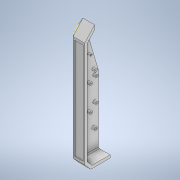
# Autodesk Inventor part: błotnik_v2
Saved by Autodesk Inventor 2022 (Build 260153000, 153)
## iProperties
Created: 2022-10-25
Part Number: błotnik_v2
Material: Generic
Document SubType Name: Modeling
Designer: Kamil
Density: 1 g/cm^3
Appearance: Default
Author: Kamil
Autodesk Inventor part; units mm, degrees
ref_plane "YZ Plane" through (0, 0, 0) normal (1, 0, 0) x (0, 1, 0)
ref_plane "XZ Plane" through (0, 0, 0) normal (0, 1, 0) x (-1, 0, 0)
ref_plane "XY Plane" through (0, 0, 0) normal (0, 0, 1) x (1, 0, 0)
sketch "Sketch1" plane through (0, 0, 0) normal (1, 0, 0) x (0, 1, 0)
  line L0 (-91.913208, 90.571897) -> (-91.913208, 0.571897)
  line L1 (-91.913208, 0.571897) -> (48.235078, 0.571897)
  arc A0 (48.235078, 0.571897) -> (67.938507, 0.571897) centre (58.086792, 2.287626) ccw
  line L2 (67.938507, 0.571897) -> (198.235078, 0.571897)
  arc A1 (198.235078, 0.571897) -> (217.938507, 0.571897) centre (208.086792, 2.287626) ccw
  line L3 (217.938507, 0.571897) -> (338.235078, 0.571897)
  arc A2 (338.235078, 0.571897) -> (357.938507, 0.571897) centre (348.086792, 2.287626) ccw
  line L4 (357.938507, 0.571897) -> (387.823998, 0.571897)
  arc A3 (387.823998, 0.571897) -> (392.823998, 1.911643) centre (387.823998, 10.571897) ccw
  line L5 (392.823998, 1.911643) -> (465.586792, 43.921262)
  arc A4 (465.586792, 43.921262) -> (453.086792, 90.571897) centre (453.086792, 65.571897) ccw
  line L6 (453.086792, 90.571897) -> (215.586792, 90.571897)
  arc A5 (215.586792, 90.571897) -> (200.586792, 90.571897) centre (208.086792, 90.571897) ccw
  line L7 (200.586792, 90.571897) -> (65.586792, 90.571897)
  arc A6 (65.586792, 90.571897) -> (50.586792, 90.571897) centre (58.086792, 90.571897) ccw
  line L8 (50.586792, 90.571897) -> (-91.913208, 90.571897)
  line L9 (394.423369, 30.080909) -> (384.836861, 44.460672)
  arc A7 (384.836916, 46.679556) -> (384.836861, 44.460672) centre (386.500961, 45.570073) ccw
  line L10 (384.836916, 46.679556) -> (394.426376, 61.062197)
  arc A8 (398.090422, 59.952509) -> (394.426376, 61.062197) centre (396.090422, 59.952714) ccw
  line L11 (398.090422, 59.952509) -> (398.08747, 31.190104)
  arc A9 (394.423369, 30.080909) -> (398.08747, 31.190104) centre (396.08747, 31.19031) ccw
  line L12 (46.086792, 47.681546) -> (11.958566, 47.681546)
  arc A10 (11.064139, 51.4704) -> (11.958566, 47.681546) centre (11.958566, 49.681546) ccw
  line L13 (11.064139, 51.4704) -> (45.192365, 68.534513)
  arc A11 (48.086792, 66.745659) -> (45.192365, 68.534513) centre (46.086792, 66.745659) ccw
  line L14 (48.086792, 66.745659) -> (48.086792, 49.681546)
  arc A12 (46.086792, 47.681546) -> (48.086792, 49.681546) centre (46.086792, 49.681546) ccw
  line L15 (278.981219, 39.534513) -> (319.328744, 19.360751)
  arc A13 (318.434316, 15.571897) -> (319.328744, 19.360751) centre (318.434316, 17.571897) ccw
  line L16 (318.434316, 15.571897) -> (237.739268, 15.571897)
  arc A14 (236.844841, 19.360751) -> (237.739268, 15.571897) centre (237.739268, 17.571897) ccw
  line L17 (236.844841, 19.360751) -> (277.192365, 39.534513)
  arc A15 (278.981219, 39.534513) -> (277.192365, 39.534513) centre (278.086792, 37.745659) ccw
  line L18 (367.833079, 75.571897) -> (388.344391, 75.571897)
  arc A16 (390.008437, 72.462414) -> (388.344391, 75.571897) centre (388.344391, 73.571897) ccw
  line L19 (390.008437, 72.462414) -> (379.752228, 57.079758)
  arc A17 (376.424082, 57.07984) -> (379.752228, 57.079758) centre (378.088183, 58.189241) ccw
  line L20 (376.424082, 57.07984) -> (366.168978, 72.462497)
  arc A18 (367.833079, 75.571897) -> (366.168978, 72.462497) centre (367.833079, 73.571897) ccw
  line L21 (361.750893, 61.061868) -> (371.338877, 46.679891)
  arc A19 (371.338822, 44.461008) -> (371.338877, 46.679891) centre (369.674777, 45.570491) ccw
  line L22 (371.338822, 44.461008) -> (361.750838, 30.080579)
  arc A20 (358.086792, 31.190063) -> (361.750838, 30.080579) centre (360.086792, 31.190063) ccw
  line L23 (358.086792, 31.190063) -> (358.086792, 59.952467)
  arc A21 (361.750893, 61.061868) -> (358.086792, 59.952467) centre (360.086792, 59.952467) ccw
  line L24 (89.12425, 75.571897) -> (177.049334, 75.571897)
  arc A22 (177.887451, 71.755978) -> (177.049334, 75.571897) centre (177.049334, 73.571897) ccw
  line L25 (177.887451, 71.755978) -> (133.924909, 51.465574)
  arc A23 (132.248676, 51.465574) -> (133.924909, 51.465574) centre (133.086792, 53.281493) ccw
  line L26 (132.248676, 51.465574) -> (88.286134, 71.755978)
  arc A24 (89.12425, 75.571897) -> (88.286134, 71.755978) centre (89.12425, 73.571897) ccw
  line L27 (-11.018781, 39.534513) -> (29.328744, 19.360751)
  arc A25 (28.434316, 15.571897) -> (29.328744, 19.360751) centre (28.434316, 17.571897) ccw
  line L28 (28.434316, 15.571897) -> (-52.260732, 15.571897)
  arc A26 (-53.155159, 19.360751) -> (-52.260732, 15.571897) centre (-52.260732, 17.571897) ccw
  line L29 (-53.155159, 19.360751) -> (-12.807635, 39.534513)
  arc A27 (-11.018781, 39.534513) -> (-12.807635, 39.534513) centre (-11.913208, 37.745659) ccw
  line L30 (117.220784, 43.755978) -> (70.924909, 22.388651)
  arc A28 (68.086792, 24.20457) -> (70.924909, 22.388651) centre (70.086792, 24.20457) ccw
  line L31 (68.086792, 24.20457) -> (68.086792, 66.939224)
  arc A29 (70.924909, 68.755143) -> (68.086792, 66.939224) centre (70.086792, 66.939224) ccw
  line L32 (70.924909, 68.755143) -> (117.220784, 47.387816)
  arc A30 (117.220784, 43.755978) -> (117.220784, 47.387816) centre (116.382668, 45.571897) ccw
  line L33 (-71.913208, 24.398135) -> (-71.913208, 66.745659)
  arc A31 (-69.018781, 68.534513) -> (-71.913208, 66.745659) centre (-69.913208, 66.745659) ccw
  line L34 (-69.018781, 68.534513) -> (-26.671256, 47.360751)
  arc A32 (-26.671256, 43.783043) -> (-26.671256, 47.360751) centre (-27.565684, 45.571897) ccw
  line L35 (-26.671256, 43.783043) -> (-69.018781, 22.60928)
  arc A33 (-71.913208, 24.398135) -> (-69.018781, 22.60928) centre (-69.913208, 24.398135) ccw
  line L36 (177.049334, 15.571897) -> (89.12425, 15.571897)
  arc A34 (88.286134, 19.387816) -> (89.12425, 15.571897) centre (89.12425, 17.571897) ccw
  line L37 (88.286134, 19.387816) -> (132.248676, 39.67822)
  arc A35 (133.924909, 39.67822) -> (132.248676, 39.67822) centre (133.086792, 37.862301) ccw
  line L38 (133.924909, 39.67822) -> (177.887451, 19.387816)
  arc A36 (177.049334, 15.571897) -> (177.887451, 19.387816) centre (177.049334, 17.571897) ccw
  line L39 (330.192365, 25.10928) -> (292.844841, 43.783043)
  arc A37 (292.844841, 47.360751) -> (292.844841, 43.783043) centre (293.739268, 45.571897) ccw
  line L40 (292.844841, 47.360751) -> (330.192365, 66.034513)
  arc A38 (333.086792, 64.245659) -> (330.192365, 66.034513) centre (331.086792, 64.245659) ccw
  line L41 (333.086792, 64.245659) -> (333.086792, 26.898135)
  arc A39 (330.192365, 25.10928) -> (333.086792, 26.898135) centre (331.086792, 26.898135) ccw
  line L42 (379.751656, 34.060723) -> (390.004607, 18.681297)
  arc A40 (388.340506, 15.571897) -> (390.004607, 18.681297) centre (388.340506, 17.571897) ccw
  line L43 (388.340506, 15.571897) -> (367.833501, 15.571897)
  arc A41 (366.169455, 18.68138) -> (367.833501, 15.571897) centre (367.833501, 17.571897) ccw
  line L44 (366.169455, 18.68138) -> (376.42351, 34.060806)
  arc A42 (379.751656, 34.060723) -> (376.42351, 34.060806) centre (378.087555, 32.951323) ccw
  line L45 (237.739268, 75.571897) -> (318.434316, 75.571897)
  arc A43 (319.328744, 71.783043) -> (318.434316, 75.571897) centre (318.434316, 73.571897) ccw
  line L46 (319.328744, 71.783043) -> (278.981219, 51.60928)
  arc A44 (277.192365, 51.60928) -> (278.981219, 51.60928) centre (278.086792, 53.398135) ccw
  line L47 (277.192365, 51.60928) -> (236.844841, 71.783043)
  arc A45 (237.739268, 75.571897) -> (236.844841, 71.783043) centre (237.739268, 73.571897) ccw
  line L48 (196.086792, 47.681546) -> (158.695156, 47.681546)
  arc A46 (157.85704, 51.497465) -> (158.695156, 47.681546) centre (158.695156, 49.681546) ccw
  line L49 (157.85704, 51.497465) -> (195.248676, 68.755143)
  arc A47 (198.086792, 66.939224) -> (195.248676, 68.755143) centre (196.086792, 66.939224) ccw
  line L50 (198.086792, 66.939224) -> (198.086792, 49.681546)
  arc A48 (196.086792, 47.681546) -> (198.086792, 49.681546) centre (196.086792, 49.681546) ccw
  line L51 (-52.260732, 75.571897) -> (28.434316, 75.571897)
  arc A49 (29.328744, 71.783043) -> (28.434316, 75.571897) centre (28.434316, 73.571897) ccw
  line L52 (29.328744, 71.783043) -> (-11.018781, 51.60928)
  arc A50 (-12.807635, 51.60928) -> (-11.018781, 51.60928) centre (-11.913208, 53.398135) ccw
  line L53 (-12.807635, 51.60928) -> (-53.155159, 71.783043)
  arc A51 (-52.260732, 75.571897) -> (-53.155159, 71.783043) centre (-52.260732, 73.571897) ccw
  line L54 (220.981219, 68.534513) -> (263.328744, 47.360751)
  arc A52 (263.328744, 43.783043) -> (263.328744, 47.360751) centre (262.434316, 45.571897) ccw
  line L55 (263.328744, 43.783043) -> (220.981219, 22.60928)
  arc A53 (218.086792, 24.398135) -> (220.981219, 22.60928) centre (220.086792, 24.398135) ccw
  line L56 (218.086792, 24.398135) -> (218.086792, 66.745659)
  arc A54 (220.981219, 68.534513) -> (218.086792, 66.745659) centre (220.086792, 66.745659) ccw
  circle A55 centre (208.086792, 2.287626) radius 2.5
  circle A56 centre (348.086792, 2.287626) radius 2.5
  circle A57 centre (243.086792, 8.071897) radius 2.5
  circle A58 centre (183.086792, 37.681546) radius 2.5
  circle A59 centre (23.086792, 37.681546) radius 2.5
  circle A60 centre (-81.913208, 83.071897) radius 2.5
  circle A61 centre (100.086792, 83.071546) radius 2.5
  circle A62 centre (260.086792, 83.071546) radius 2.5
  circle A63 centre (343.086792, 37.681546) radius 2.5
  circle A64 centre (348.086792, 83.071897) radius 2.5
  circle A65 centre (58.086792, 2.287626) radius 2.5
  circle A66 centre (-81.913208, 8.071897) radius 2.5
  line L57 (413.086792, 68.571897) -> (453.086792, 68.571897)
  arc A67 (453.086792, 62.571897) -> (453.086792, 68.571897) centre (453.086792, 65.571897) ccw
  line L58 (453.086792, 62.571897) -> (413.086792, 62.571897)
  arc A68 (413.086792, 68.571897) -> (413.086792, 62.571897) centre (413.086792, 65.571897) ccw
  line L59 (493.086792, 110.571897) -> (493.086792, -89.428103)
  line L60 (493.086792, -89.428103) -> (-191.913208, -89.428103)
  circle A69 centre (453.086792, 65.571897) radius 40
  circle A70 centre (-151.913208, 65.571897) radius 40
  line L61 (493.086792, -89.428103) -> (-191.913208, -89.428103)
  line L62 (-191.913208, -89.428103) -> (-191.913208, -23.428103)
  line L63 (-191.913208, -23.428103) -> (493.086792, -23.428103)
  line L64 (493.086792, -23.428103) -> (493.086792, -89.428103)
  line L65 (493.086792, -89.428103) -> (513.086792, -89.428103)
  line L66 (493.086792, 111.079815) -> (493.086792, -89.428103)
  line L67 (453.086792, 65.571897) -> (503.100187, 121.461612)
  line L68 (479.760603, 95.379745) -> (493.097508, 110.283669)
  line L69 (493.097508, 110.283669) -> (453.663093, 145.571897)
  line L70 (453.663093, 145.571897) -> (531.887738, 75.571897)
  line L71 (-151.913208, 65.571897) -> (-191.775038, 110.416456)
  line L72 (-178.487761, 95.46827) -> (-191.775038, 110.416456)
  line L73 (-191.775038, 110.416456) -> (-234.945881, 72.042373)
  line L74 (-234.945881, 72.042373) -> (-158.179562, 140.279101)
  line L75 (528.008583, -89.357621) -> (513.008583, -89.357621)
  line L76 (518.005904, 87.994176) -> (528.008583, 99.17212)
  line L77 (465.586792, 134.901872) -> (475.589471, 146.079815)
  line L78 (532.147616, 95.46827) -> (475.589471, 146.079815)
  line L79 (475.589471, 146.079815) -> (554.381712, 75.571897)
  line L80 (518.005904, 87.994176) -> (531.887738, 75.571897)
  line L81 (543.062687, 75.571897) -> (584.645568, 75.571897)
  line L82 (584.645568, 75.571897) -> (398.349618, 75.571897)
  line L83 (-158.179562, 140.279101) -> (-132.743704, 162.756041)
  line L84 (-226.991417, -89.357621) -> (-211.991417, -89.357621)
  line L85 (-250.129793, 130.571897) -> (-250.129793, 145.571897)
  line L86 (-191.913208, -89.428103) -> (-191.913208, 65.571897)
  line L87 (-191.913208, 110.293639) -> (-191.913208, 110.571897)
  line L88 (-191.913208, 110.293639) -> (-201.878665, 121.504778)
  line L89 (-201.888524, 121.496015) -> (-174.803157, 145.571897)
  line L90 (-201.888524, 121.496015) -> (-254.656636, 74.591027)
  line L91 (-211.913208, -4.093976) -> (-211.913208, 29.447632)
  line L92 (-191.913208, 29.447632) -> (-191.913208, -4.093976)
  line L93 (-226.913208, -4.093976) -> (-226.913208, 29.447632)
  line L94 (-211.913208, 29.447632) -> (-211.913208, -4.093976)
  line L95 (-226.913208, -4.093976) -> (-211.913208, -4.093976)
  line L96 (-211.913208, -4.093976) -> (-211.913208, 115.899208)
  line L97 (-211.913208, 115.899208) -> (-226.913208, 115.899208)
  line L98 (-226.913208, 115.899208) -> (-226.913208, -4.093976)
  line L99 (-226.913208, -4.093976) -> (-211.913208, -4.093976)
  line L100 (-211.913208, -4.093976) -> (-211.913208, -158.327462)
  line L101 (-211.913208, -158.327462) -> (-226.913208, -158.327462)
  line L102 (-226.913208, -158.327462) -> (-226.913208, -4.093976)
  line L103 (531.887738, 75.571897) -> (543.890953, 88.985429)
  line L104 (-191.913208, 110.293639) -> (-203.871757, 123.747006)
  line L105 (-211.913208, -4.093976) -> (-229.913208, -4.093976)
  line L106 (-229.913208, -4.093976) -> (-229.913208, 127.927783)
  line L107 (-229.913208, 127.927783) -> (-229.913208, -180.474457)
  line L108 (-203.871757, 123.747006) -> (-168.215619, 155.441351)
  line L109 (-168.215619, 155.441351) -> (-240.454048, 91.229415)
  line L110 (543.890953, 88.985429) -> (459.90651, 164.139633)
  line L111 (459.90651, 164.139633) -> (563.854127, 71.121209)
  circle A71 centre (348.086792, 83.071897) radius 6.710252
  circle A72 centre (-81.913208, 8.071897) radius 5.766352
  line L112 (-211.913208, -23.428103) -> (-229.913208, -23.428103)
  line L113 (493.086792, -23.428103) -> (732.784985, -23.428103)
  line L114 (558.880507, 75.571897) -> (222.333079, -23.428103)
  line L115 (222.333079, -23.428103) -> (-229.913208, -23.428103)
  line L116 (453.086792, 105.571897) -> (495.489419, 105.571897)
  line L117 (453.086792, 105.571897) -> (453.086792, 123.571897)
  line L118 (453.086792, 123.571897) -> (517.1971, 123.571897)
  line L119 (453.086792, 123.571897) -> (453.086792, 138.571897)
  line L120 (453.086792, 138.571897) -> (512.645416, 138.571897)
  line L121 (453.086792, 138.571897) -> (-211.913208, 138.571897)
  line L122 (453.086792, 123.571897) -> (-280.749903, 123.571897)
  point P0 (0, 0)
  point P1 (0, 0)
  point P2 (558.880507, 75.571897)
  point P3 (488.478326, 138.571897)
  point P4 (-187.193755, 138.571897)
  point P5 (-203.716104, 123.571897)
  point P6 (-204.068755, 123.571897)
  point P7 (-229.913208, 100.59905)
  point P8 (-211.913208, 92.515861)
  point P9 (-176.975167, 123.571897)
  point P10 (478.247981, 123.571897)
  point P11 (493.086792, 110.293259)
  point P12 (493.086792, 110.271694)
  dimension "d2" = 685
  dimension "d3" = 200
  dimension "d9" = 20
  dimension "d11" = 20
  dimension "d13" = 15
  dimension "d14" = 15
  dimension "d15" = 15
  dimension "d20" = 15
  dimension "d23" = 18
  dimension "d25" = 18
  dimension "d26" = 18
  dimension "d28" = 18
  dimension "d29" = 15
  constraints: 246 end point, 118 point on circle, 73 centre point, 26 point on line, 17 perpendicular, 12 parallel, 7 horizontal, 3 coincident, 3 tangent, 2 vertical, 1 collinear
  measures "d2" distance of L59.start L87.end
  measures "d3" distance of L59.start L59.end
  measures "d9" distance of L68.start L68.end
  measures "d11" distance of L71.end L72.start
  measures "d13" distance of L75.start L75.end
  measures "d14" distance of L76.start L76.end
  measures "d15" distance of L77.end L77.start
  measures "d20" distance of L87.start L88.end
  measures "d23" distance of L70.end L103.end
  measures "d25" distance of L87.start L104.end
  measures "d26" distance of L99.end L105.end
  measures "d28" distance of L116.start L117.end
  measures "d29" distance of L117.end L119.end
extrude "Extrusion1" add sketch "Sketch1" along normal blind 100 contours L119 L120 L69 L118 | L122 L74 L121 L119 | L118 L78 L67 L69 | L69 L77 L120 L78 L118 | L122 L89 L121 L74 | L74 L73 L88 L89 L122 | L112 L102 L95 L100 | L67 L78 L76 L70 | L69 L120 L77 | L118 L110 L103 L79 L78 | L78 L120 L110 L118 | L122 L104 L108 L121 L89 | L89 L104 L122 | L95 L93 L98 L73 L96 L91 | L112 L107 L105 L102 | L81 L79 L103 L111 | L103 L79 L81 L82 | L70 L76 L78 L79 L103 | L73 L96 L90 L89 L88 | L89 L90 L96 L97 L109 L122 L104 | L105 L106 L73 L98 L93 | L73 L98 L90 L96 | L73 L106 L90 L98 | L90 L98 L109 L97 L96 | L90 L106 L109 L98
extrude "Extrusion2" add sketch "Sketch1" against normal blind 20 contours L8 A6 L7 A5 L6 A69 L57 A68 L58 L114 L42 A42 L44 L3 A1 L2 A0 L1 L0 | L0 L1 A0 L2 A1 L3 L114 L63 L86 A70 L71 L74 L122 L117 A69 L6 A5 L7 A6 L8 | A69 L67 A4 L6 | L6 A4 L67 L82 A69 | L116 L67 A69 | L117 L118 L69 L59 L67 L116 | L82 L67 A67 L57 A69 | L44 A42 L42 L114 | L67 A69 L82 A4 | A4 L82 L67 | L67 L116 L59 L82 A69 | L67 L59 L116 | L119 L120 L69 L118 | L122 L74 L121 L119 | A69 L58 A68 L57 | L57 A67 L58 A69 | L82 A4 L114 A69 L58 A67 L67 | L115 L100 L91 L96 L73 L71 A70 L86 | L82 A69 L114 A4 | L82 L59 A69 | L67 L70 L82 L59 | L118 L78 L67 L69 | L69 L77 L120 L78 L118 | L122 L89 L121 L74 | L74 L73 L88 L89 L122 | L112 L102 L95 L100 | L114 A69 L59 | L59 L82 L81 L114 | L67 L78 L76 L70 | L69 L120 L77 | L118 L110 L103 L79 L78 | L78 L120 L110 L118 | L122 L104 L108 L121 L89 | L89 L104 L122 | L95 L93 L98 L73 L96 L91 | L112 L107 L105 L102 | L81 L79 L103 L111 | L103 L79 L81 L82 | L70 L76 L78 L79 L103 | A70 | L73 L96 L90 L89 L88 | L89 L90 L96 L97 L109 L122 L104 | L122 L109 L104 | L105 L106 L73 L98 L93 | L73 L98 L90 L96 | L73 L106 L90 L98 | L90 L98 L109 L97 L96 | L90 L106 L109 L98 | L9 A7 L10 A8 L11 A9 | L12 A10 L13 A11 L14 A12 | L15 A13 L16 A14 L17 A15 | L18 A16 L19 A17 L20 A18 | L21 A19 L22 A20 L23 A21 | L24 A22 L25 A23 L26 A24 | L27 A25 L28 A26 L29 A27 | L30 A28 L31 A29 L32 A30 | L33 A31 L34 A32 L35 A33 | L36 A34 L37 A35 L38 A36 | L39 A37 L40 A38 L41 A39 | L45 A43 L46 A44 L47 A45 | L48 A46 L49 A47 L50 A48 | L51 A49 L52 A50 L53 A51 | L54 A52 L55 A53 L56 A54 | A55 | A57 | A58 | A59 | A60 | A61 | A62 | A63 | A65
chamfer "Chamfer1" distance 20 angle 45 6 edges at (-20, 523.6794, 107.0719) (-20, 390.6068, 26.0719) (-20, -3.7901, -23.4281) (-20, 150.6423, 138.5719) (-20, -208.5535, 119.5855) (-20, -229.9132, 38.5855)
sketch "Sketch2" plane through (100, 0, 0) normal (1, 0, 0) x (0, 0, -1)
  line L0 (-123.571897, 478.247981) -> (-75.571897, 531.887738)
  line L1 (-75.571897, 531.887738) -> (-75.571897, 558.880507)
  line L2 (-75.571897, 558.880507) -> (-138.571897, 488.478326)
  line L3 (-138.571897, 488.478326) -> (-138.571897, -187.193755)
  line L4 (-138.571897, -187.193755) -> (-123.747006, -203.871757)
  line L5 (-123.747006, -203.871757) -> (-123.571897, -203.716104)
  line L6 (-123.571897, -203.716104) -> (-123.571897, -204.068755)
  line L7 (-123.571897, -204.068755) -> (-100.59905, -229.913208)
  line L8 (-100.59905, -229.913208) -> (23.428103, -229.913208)
  line L9 (23.428103, -229.913208) -> (23.428103, -211.913208)
  line L10 (23.428103, -211.913208) -> (-92.515861, -211.913208)
  line L11 (-92.515861, -211.913208) -> (-123.571897, -176.975167)
  line L12 (-123.571897, -176.975167) -> (-123.571897, 478.247981)
  line L13 (-123.571897, -203.716104) -> (-123.571897, -204.068755)
  line L14 (-123.747006, -203.871757) -> (-123.571897, -204.068755)
  point P0 (0, 0)
  constraints: 2 end point
extrude "Extrusion3" add sketch "Sketch2" against normal up to surface (100 mm away) contours L5 L6 L14
chamfer "Chamfer2" distance 6 angle 45 4 edges at (0, -211.9132, 34.5439) (0, -194.4442, 108.0439) (0, 150.6364, 123.5719) (0, 512.4926, 92.9278)
chamfer "Chamfer3" distance 6 angle 45 1 edges at (0, 489.0199, 113.9326)
sketch "Sketch3" plane through (100, -187.193755, 138.571897) normal (0, 0, 1) x (1, 0, 0)
  line L0 (-100, 0) -> (-100, 675.672081)
  line L1 (-100, 0) -> (0, 0)
  line L2 (0, 675.672081) -> (0, 0)
  line L3 (-100, 675.672081) -> (0, 675.672081)
  line L4 (-100, 0) -> (-25, 0)
  line L5 (-25, 0) -> (-25, 62.127506)
  line L6 (-25, 62.127506) -> (-100, 62.127506)
  line L7 (-100, 62.127506) -> (-100, 0)
  line L8 (-100, -42.719453) -> (0, -42.719453)
  line L9 (-25, -42.719453) -> (80.994061, -42.719453)
  line L10 (80.994061, -42.719453) -> (80.994061, 814.152371)
  line L11 (80.994061, 814.152371) -> (-25, 814.152371)
  line L12 (-25, 814.152371) -> (-25, -42.719453)
  point P0 (-100, 187.193755)
  dimension "d45" = 75
  constraints: 16 end point, 4 parallel, 2 horizontal, 2 perpendicular, 2 point on line
  measures "d45" distance of L6.end L5.end
extrude "Extrusion4" cut sketch "Sketch3" against normal through all contours L5 L12 L3 L2 L1 | L1 L2 L3 L12 L11 L10 L9 L8
sketch "Sketch4" plane through (0, 0, 0) normal (1, 0, 0) x (0, 0, -1)
  line L0 (-117.571897, 475.955362) -> (-75.571897, 522.890149)
  line L1 (-117.571897, -174.693971) -> (-117.571897, 475.955362)
  line L2 (-89.821464, -205.913208) -> (-117.571897, -174.693971)
  line L3 (23.428103, -205.913208) -> (-89.821464, -205.913208)
  line L4 (23.428103, -205.913208) -> (23.428103, 222.333079)
  line L5 (23.428103, 222.333079) -> (-75.571897, 558.880507)
  line L6 (-75.571897, 522.890149) -> (-75.571897, 558.880507)
  circle A0 centre (-8.071897, -81.913208) radius 5.766352
  circle A1 centre (-83.071897, 348.086792) radius 6.710252
  circle A2 centre (-8.071897, -81.913208) radius 11.228159
  circle A3 centre (-83.071897, 348.086792) radius 6.710252
  circle A4 centre (-83.071897, 348.086792) radius 15.329572
  point P0 (0, 0)
  constraints: 2 centre point, 2 coincident
extrude "Extrusion5" add sketch "Sketch4" along normal blind 15 contours A2 | A4
sketch "Sketch5" plane through (0, -187.193755, 138.571897) normal (0, 0, 1) x (1, 0, 0)
  line L0 (75, 0) -> (75, 675.672081)
  line L1 (0, 675.672081) -> (75, 675.672081)
  line L2 (0, 0) -> (0, 675.672081)
  line L3 (0, 0) -> (75, 0)
  line L4 (10, 71.808614) -> (65, 71.808614)
  line L5 (65, 71.808614) -> (65, 16)
  line L6 (65, 16) -> (10, 16)
  line L7 (10, 16) -> (10, 71.808614)
  line L8 (75, 665.441736) -> (75, 10.218588)
  line L9 (0, 0) -> (75, 0)
  line L10 (75, 0) -> (75, 16)
  line L11 (75, 16) -> (0, 16)
  line L12 (0, 16) -> (0, 0)
  line L13 (75, 337.830162) -> (0, 337.82445)
  line L14 (0, 12.499784) -> (0, 663.149116)
  line L15 (10, 71.808614) -> (65, 71.808614)
  line L16 (65, 71.808614) -> (65, 325.25114)
  line L17 (65, 325.25114) -> (10, 325.25114)
  line L18 (10, 325.25114) -> (10, 71.808614)
  line L19 (0, 675.672081) -> (75, 675.672081)
  line L20 (75, 675.672081) -> (75, 659.672081)
  line L21 (75, 659.672081) -> (0, 659.672081)
  line L22 (0, 659.672081) -> (0, 675.672081)
  line L23 (10, 325.25114) -> (65, 325.25114)
  line L24 (65, 325.25114) -> (65, 659.672081)
  line L25 (65, 659.672081) -> (10, 659.672081)
  line L26 (10, 659.672081) -> (10, 325.25114)
  line L27 (10, 348.678223) -> (10, 311.259118)
  point P0 (0, 187.193755)
  point P1 (37.5, 16)
  point P2 (37.5, 16)
  point P3 (10, 325.25114)
  point P4 (65, 71.808614)
  point P5 (10, 659.672081)
  dimension "d50" = 55
  dimension "d51" = 16
  dimension "d52" = 16
  constraints: 44 end point, 10 parallel, 5 horizontal, 5 perpendicular, 5 point on line, 4 midpoint
  measures "d50" distance of L5.end L6.end
  measures "d51" distance of L10.end L9.end
  measures "d52" distance of L19.end L20.end
extrude "Extrusion6" cut sketch "Sketch5" against normal blind 4 contours L6 L7 L4 L5 | L24 L17 L26 L13 | L13 L26 L21 L24 | L4 L18 L17 L16
sketch "Sketch6" plane through (0, 0, 0) normal (1, 0, 0) x (0, 0, -1)
  circle A0 centre (-83.071897, -81.913208) radius 2.5
  circle A1 centre (-83.071897, -81.913208) radius 9.579243
  circle A2 centre (-83.071897, -81.913208) radius 3.982144
  point P0 (0, 0)
  constraints: 2 centre point, 2 coincident
extrude "Extrusion7" add sketch "Sketch6" along normal up to surface (15 mm away) contours A1
sketch "Sketch7" plane through (0, 0, 0) normal (1, 0, 0) x (0, 0, -1)
  circle A0 centre (-37.681546, 343.086792) radius 2.5
  circle A1 centre (-37.681546, 343.086792) radius 3
  circle A2 centre (-37.681546, 343.086792) radius 7.013487
  point P0 (0, 0)
  dimension "d57" = 6
  constraints: 2 centre point, 2 coincident
  measures "d57" diameter of A1
extrude "Extrusion8" add sketch "Sketch7" along normal up to surface (15 mm away) contours A2
sketch "Sketch8" plane through (-20, 0, 0) normal (-1, 0, 0) x (0, 0, 1)
  circle A0 centre (8.071897, -81.913208) radius 5.766352
  circle A1 centre (83.071897, 348.086792) radius 6.710252
  line L0 (91.617729, -209.913208) -> (-3.428103, -209.913208)
  line L1 (118.571897, -179.589768) -> (91.617729, -209.913208)
  line L2 (118.571897, 480.83626) -> (118.571897, -179.589768)
  line L3 (84.621787, 518.775335) -> (118.571897, 480.83626)
  line L4 (-3.428103, 219.452466) -> (84.621787, 518.775335)
  line L5 (-3.428103, -209.913208) -> (-3.428103, 219.452466)
  point P0 (0, 0)
sketch "Sketch9" plane through (-20, 0, 0) normal (-1, 0, 0) x (0, 0, 1)
  line L0 (90.571897, -91.913208) -> (0.571897, -91.913208)
  line L1 (0.571897, -91.913208) -> (0.571897, 48.235078)
  arc A0 (0.571897, 67.938507) -> (0.571897, 48.235078) centre (2.287626, 58.086792) ccw
  line L2 (0.571897, 67.938507) -> (0.571897, 198.235078)
  arc A1 (0.571897, 217.938507) -> (0.571897, 198.235078) centre (2.287626, 208.086792) ccw
  line L3 (0.571897, 217.938507) -> (0.571897, 338.235078)
  arc A2 (0.571897, 357.938507) -> (0.571897, 338.235078) centre (2.287626, 348.086792) ccw
  line L4 (0.571897, 357.938507) -> (0.571897, 387.823998)
  arc A3 (1.911643, 392.823998) -> (0.571897, 387.823998) centre (10.571897, 387.823998) ccw
  line L5 (1.911643, 392.823998) -> (43.921262, 465.586792)
  arc A4 (90.571897, 453.086792) -> (43.921262, 465.586792) centre (65.571897, 453.086792) ccw
  line L6 (90.571897, 453.086792) -> (90.571897, 215.586792)
  arc A5 (90.571897, 200.586792) -> (90.571897, 215.586792) centre (90.571897, 208.086792) ccw
  line L7 (90.571897, 200.586792) -> (90.571897, 65.586792)
  arc A6 (90.571897, 50.586792) -> (90.571897, 65.586792) centre (90.571897, 58.086792) ccw
  line L8 (90.571897, 50.586792) -> (90.571897, -91.913208)
  line L9 (30.080909, 394.423369) -> (44.460672, 384.836861)
  arc A7 (44.460672, 384.836861) -> (46.679556, 384.836916) centre (45.570073, 386.500961) ccw
  line L10 (46.679556, 384.836916) -> (61.062197, 394.426376)
  arc A8 (61.062197, 394.426376) -> (59.952509, 398.090422) centre (59.952714, 396.090422) ccw
  line L11 (59.952509, 398.090422) -> (31.190104, 398.08747)
  arc A9 (31.190104, 398.08747) -> (30.080909, 394.423369) centre (31.19031, 396.08747) ccw
  line L12 (47.681546, 46.086792) -> (47.681546, 11.958566)
  arc A10 (47.681546, 11.958566) -> (51.4704, 11.064139) centre (49.681546, 11.958566) ccw
  line L13 (51.4704, 11.064139) -> (68.534513, 45.192365)
  arc A11 (68.534513, 45.192365) -> (66.745659, 48.086792) centre (66.745659, 46.086792) ccw
  line L14 (66.745659, 48.086792) -> (49.681546, 48.086792)
  arc A12 (49.681546, 48.086792) -> (47.681546, 46.086792) centre (49.681546, 46.086792) ccw
  line L15 (39.534513, 278.981219) -> (19.360751, 319.328744)
  arc A13 (19.360751, 319.328744) -> (15.571897, 318.434316) centre (17.571897, 318.434316) ccw
  line L16 (15.571897, 318.434316) -> (15.571897, 237.739268)
  arc A14 (15.571897, 237.739268) -> (19.360751, 236.844841) centre (17.571897, 237.739268) ccw
  line L17 (19.360751, 236.844841) -> (39.534513, 277.192365)
  arc A15 (39.534513, 277.192365) -> (39.534513, 278.981219) centre (37.745659, 278.086792) ccw
  line L18 (75.571897, 367.833079) -> (75.571897, 388.344391)
  arc A16 (75.571897, 388.344391) -> (72.462414, 390.008437) centre (73.571897, 388.344391) ccw
  line L19 (72.462414, 390.008437) -> (57.079758, 379.752228)
  arc A17 (57.079758, 379.752228) -> (57.07984, 376.424082) centre (58.189241, 378.088183) ccw
  line L20 (57.07984, 376.424082) -> (72.462497, 366.168978)
  arc A18 (72.462497, 366.168978) -> (75.571897, 367.833079) centre (73.571897, 367.833079) ccw
  line L21 (61.061868, 361.750893) -> (46.679891, 371.338877)
  arc A19 (46.679891, 371.338877) -> (44.461008, 371.338822) centre (45.570491, 369.674777) ccw
  line L22 (44.461008, 371.338822) -> (30.080579, 361.750838)
  arc A20 (30.080579, 361.750838) -> (31.190063, 358.086792) centre (31.190063, 360.086792) ccw
  line L23 (31.190063, 358.086792) -> (59.952467, 358.086792)
  arc A21 (59.952467, 358.086792) -> (61.061868, 361.750893) centre (59.952467, 360.086792) ccw
  line L24 (75.571897, 89.12425) -> (75.571897, 177.049334)
  arc A22 (75.571897, 177.049334) -> (71.755978, 177.887451) centre (73.571897, 177.049334) ccw
  line L25 (71.755978, 177.887451) -> (51.465574, 133.924909)
  arc A23 (51.465574, 133.924909) -> (51.465574, 132.248676) centre (53.281493, 133.086792) ccw
  line L26 (51.465574, 132.248676) -> (71.755978, 88.286134)
  arc A24 (71.755978, 88.286134) -> (75.571897, 89.12425) centre (73.571897, 89.12425) ccw
  line L27 (39.534513, -11.018781) -> (19.360751, 29.328744)
  arc A25 (19.360751, 29.328744) -> (15.571897, 28.434316) centre (17.571897, 28.434316) ccw
  line L28 (15.571897, 28.434316) -> (15.571897, -52.260732)
  arc A26 (15.571897, -52.260732) -> (19.360751, -53.155159) centre (17.571897, -52.260732) ccw
  line L29 (19.360751, -53.155159) -> (39.534513, -12.807635)
  arc A27 (39.534513, -12.807635) -> (39.534513, -11.018781) centre (37.745659, -11.913208) ccw
  line L30 (43.755978, 117.220784) -> (22.388651, 70.924909)
  arc A28 (22.388651, 70.924909) -> (24.20457, 68.086792) centre (24.20457, 70.086792) ccw
  line L31 (24.20457, 68.086792) -> (66.939224, 68.086792)
  arc A29 (66.939224, 68.086792) -> (68.755143, 70.924909) centre (66.939224, 70.086792) ccw
  line L32 (68.755143, 70.924909) -> (47.387816, 117.220784)
  arc A30 (47.387816, 117.220784) -> (43.755978, 117.220784) centre (45.571897, 116.382668) ccw
  line L33 (24.398135, -71.913208) -> (66.745659, -71.913208)
  arc A31 (66.745659, -71.913208) -> (68.534513, -69.018781) centre (66.745659, -69.913208) ccw
  line L34 (68.534513, -69.018781) -> (47.360751, -26.671256)
  arc A32 (47.360751, -26.671256) -> (43.783043, -26.671256) centre (45.571897, -27.565684) ccw
  line L35 (43.783043, -26.671256) -> (22.60928, -69.018781)
  arc A33 (22.60928, -69.018781) -> (24.398135, -71.913208) centre (24.398135, -69.913208) ccw
  line L36 (15.571897, 177.049334) -> (15.571897, 89.12425)
  arc A34 (15.571897, 89.12425) -> (19.387816, 88.286134) centre (17.571897, 89.12425) ccw
  line L37 (19.387816, 88.286134) -> (39.67822, 132.248676)
  arc A35 (39.67822, 132.248676) -> (39.67822, 133.924909) centre (37.862301, 133.086792) ccw
  line L38 (39.67822, 133.924909) -> (19.387816, 177.887451)
  arc A36 (19.387816, 177.887451) -> (15.571897, 177.049334) centre (17.571897, 177.049334) ccw
  line L39 (25.10928, 330.192365) -> (43.783043, 292.844841)
  arc A37 (43.783043, 292.844841) -> (47.360751, 292.844841) centre (45.571897, 293.739268) ccw
  line L40 (47.360751, 292.844841) -> (66.034513, 330.192365)
  arc A38 (66.034513, 330.192365) -> (64.245659, 333.086792) centre (64.245659, 331.086792) ccw
  line L41 (64.245659, 333.086792) -> (26.898135, 333.086792)
  arc A39 (26.898135, 333.086792) -> (25.10928, 330.192365) centre (26.898135, 331.086792) ccw
  line L42 (34.060723, 379.751656) -> (18.681297, 390.004607)
  arc A40 (18.681297, 390.004607) -> (15.571897, 388.340506) centre (17.571897, 388.340506) ccw
  line L43 (15.571897, 388.340506) -> (15.571897, 367.833501)
  arc A41 (15.571897, 367.833501) -> (18.68138, 366.169455) centre (17.571897, 367.833501) ccw
  line L44 (18.68138, 366.169455) -> (34.060806, 376.42351)
  arc A42 (34.060806, 376.42351) -> (34.060723, 379.751656) centre (32.951323, 378.087555) ccw
  line L45 (75.571897, 237.739268) -> (75.571897, 318.434316)
  arc A43 (75.571897, 318.434316) -> (71.783043, 319.328744) centre (73.571897, 318.434316) ccw
  line L46 (71.783043, 319.328744) -> (51.60928, 278.981219)
  arc A44 (51.60928, 278.981219) -> (51.60928, 277.192365) centre (53.398135, 278.086792) ccw
  line L47 (51.60928, 277.192365) -> (71.783043, 236.844841)
  arc A45 (71.783043, 236.844841) -> (75.571897, 237.739268) centre (73.571897, 237.739268) ccw
  line L48 (47.681546, 196.086792) -> (47.681546, 158.695156)
  arc A46 (47.681546, 158.695156) -> (51.497465, 157.85704) centre (49.681546, 158.695156) ccw
  line L49 (51.497465, 157.85704) -> (68.755143, 195.248676)
  arc A47 (68.755143, 195.248676) -> (66.939224, 198.086792) centre (66.939224, 196.086792) ccw
  line L50 (66.939224, 198.086792) -> (49.681546, 198.086792)
  arc A48 (49.681546, 198.086792) -> (47.681546, 196.086792) centre (49.681546, 196.086792) ccw
  line L51 (75.571897, -52.260732) -> (75.571897, 28.434316)
  arc A49 (75.571897, 28.434316) -> (71.783043, 29.328744) centre (73.571897, 28.434316) ccw
  line L52 (71.783043, 29.328744) -> (51.60928, -11.018781)
  arc A50 (51.60928, -11.018781) -> (51.60928, -12.807635) centre (53.398135, -11.913208) ccw
  line L53 (51.60928, -12.807635) -> (71.783043, -53.155159)
  arc A51 (71.783043, -53.155159) -> (75.571897, -52.260732) centre (73.571897, -52.260732) ccw
  line L54 (68.534513, 220.981219) -> (47.360751, 263.328744)
  arc A52 (47.360751, 263.328744) -> (43.783043, 263.328744) centre (45.571897, 262.434316) ccw
  line L55 (43.783043, 263.328744) -> (22.60928, 220.981219)
  arc A53 (22.60928, 220.981219) -> (24.398135, 218.086792) centre (24.398135, 220.086792) ccw
  line L56 (24.398135, 218.086792) -> (66.745659, 218.086792)
  arc A54 (66.745659, 218.086792) -> (68.534513, 220.981219) centre (66.745659, 220.086792) ccw
  circle A55 centre (2.287626, 208.086792) radius 2.5
  circle A56 centre (2.287626, 348.086792) radius 2.5
  circle A57 centre (8.071897, 243.086792) radius 2.5
  circle A58 centre (37.681546, 183.086792) radius 2.5
  circle A59 centre (37.681546, 23.086792) radius 2.5
  circle A60 centre (83.071897, -81.913208) radius 2.5
  circle A61 centre (83.071546, 100.086792) radius 2.5
  circle A62 centre (83.071546, 260.086792) radius 2.5
  circle A63 centre (37.681546, 343.086792) radius 2.5
  circle A64 centre (83.071897, 348.086792) radius 2.5
  circle A65 centre (2.287626, 58.086792) radius 2.5
  circle A66 centre (8.071897, -81.913208) radius 2.5
  line L57 (68.571897, 413.086792) -> (68.571897, 453.086792)
  arc A67 (68.571897, 453.086792) -> (62.571897, 453.086792) centre (65.571897, 453.086792) ccw
  line L58 (62.571897, 453.086792) -> (62.571897, 413.086792)
  arc A68 (62.571897, 413.086792) -> (68.571897, 413.086792) centre (65.571897, 413.086792) ccw
  circle A69 centre (37.681546, 343.086792) radius 3
  circle A70 centre (37.681546, 343.086792) radius 3
  circle A71 centre (83.071546, 260.086792) radius 3
  circle A72 centre (37.681546, 183.086792) radius 3
  circle A73 centre (2.287626, 208.086792) radius 3
  circle A74 centre (2.287626, 58.086792) radius 3
  circle A75 centre (83.071546, 100.086792) radius 3
  circle A76 centre (83.071897, -81.913208) radius 3.982144
  circle A77 centre (83.071897, -81.913208) radius 3.982144
  circle A78 centre (37.681546, 23.086792) radius 3
  point P0 (0, 0)
  dimension "d60" = 6
  dimension "d61" = 6
  dimension "d62" = 6
  dimension "d63" = 6
  dimension "d64" = 6
  dimension "d65" = 6
  constraints: 8 centre point, 8 coincident
  measures "d60" diameter of A71
  measures "d61" diameter of A72
  measures "d62" diameter of A73
  measures "d63" diameter of A74
  measures "d64" diameter of A75
  measures "d65" diameter of A78
extrude "Extrusion9" cut sketch "Sketch9" against normal through all contours A55 | A57 | A58 | A59 | A60 | A61 | A62 | A63 | A65 | A66 | A69 | A71 | A72 | A73 | A74 | A75 | A76 | A78
sketch "Sketch10" plane through (0, 0, 0) normal (1, 0, 0) x (0, 0, -1)
  circle A0 centre (-8.071897, 243.086792) radius 2.5
  circle A1 centre (-2.287626, 58.086792) radius 3
  circle A2 centre (-83.071546, 100.086792) radius 3
  circle A3 centre (-83.071546, 260.086792) radius 3
  circle A4 centre (-2.287626, 208.086792) radius 3
  circle A5 centre (-37.681546, 23.086792) radius 3
  circle A6 centre (-37.681546, 183.086792) radius 3
  circle A7 centre (-83.071897, -81.913208) radius 9.579243
  circle A8 centre (-83.071897, 348.086792) radius 15.329572
  circle A9 centre (-8.071897, -81.913208) radius 11.228159
  line L0 (-117.571897, 475.955362) -> (-75.571897, 522.890149)
  line L1 (-117.571897, -174.693971) -> (-117.571897, 475.955362)
  line L2 (-89.821464, -205.913208) -> (-117.571897, -174.693971)
  line L3 (23.428103, -205.913208) -> (-89.821464, -205.913208)
  line L4 (23.428103, -205.913208) -> (23.428103, 222.333079)
  line L5 (23.428103, 222.333079) -> (-75.571897, 558.880507)
  line L6 (-75.571897, 522.890149) -> (-75.571897, 558.880507)
  circle A10 centre (-37.681546, 343.086792) radius 7.013487
  circle A11 centre (-37.681546, 23.086792) radius 3
  circle A12 centre (-37.681546, 23.086792) radius 10
  circle A13 centre (-83.071546, 100.086792) radius 3
  circle A14 centre (-83.071546, 100.086792) radius 10
  circle A15 centre (-2.287626, 58.086792) radius 3
  circle A16 centre (-2.287626, 58.086792) radius 10
  circle A17 centre (-37.681546, 183.086792) radius 3
  circle A18 centre (-37.681546, 183.086792) radius 10
  circle A19 centre (-2.287626, 208.086792) radius 3
  circle A20 centre (-2.287626, 208.086792) radius 10
  circle A21 centre (-83.071546, 260.086792) radius 10
  circle A22 centre (-8.071897, 243.086792) radius 10
  point P0 (0, 0)
  dimension "d68" = 20
  dimension "d69" = 20
  dimension "d70" = 20
  dimension "d71" = 20
  dimension "d72" = 20
  dimension "d73" = 20
  dimension "d74" = 20
  constraints: 7 centre point, 7 coincident
  measures "d68" diameter of A12
  measures "d69" diameter of A14
  measures "d70" diameter of A16
  measures "d71" diameter of A18
  measures "d72" diameter of A20
  measures "d73" diameter of A21
  measures "d74" diameter of A22
extrude "Extrusion10" add sketch "Sketch10" along normal blind 15 contours A12 | A14 | A16 | A18 | A20 | A21 | A22
body "Solid1"
